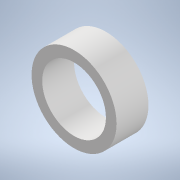
# Autodesk Inventor part: 3mmSpacer
Saved by Autodesk Inventor 2022 (Build 260153000, 153)
## iProperties
Created: 2023-09-19
Part Number: 3mmSpacer
Material: Generic
Document SubType Name: Modeling
Designer: THK
Density: 1 g/cm^3
Appearance: Default
Author: THK
Autodesk Inventor part; units mm, degrees
ref_plane "YZ Plane" through (0, 0, 0) normal (1, 0, 0) x (0, 1, 0)
ref_plane "XZ Plane" through (0, 0, 0) normal (0, 1, 0) x (-1, 0, 0)
ref_plane "XY Plane" through (0, 0, 0) normal (0, 0, 1) x (1, 0, 0)
sketch "Sketch1" plane through (0, 0, 0) normal (0, 0, 1) x (1, 0, 0)
  circle A0 centre (0, 0) radius 3
  circle A1 centre (0, 0) radius 4
  dimension "d0" = 6
  dimension "d1" = 8
  constraints: 2 centre point, 2 coincident
  measures "d0" diameter of A0
  measures "d1" diameter of A1
extrude "Extrusion1" add sketch "Sketch1" along normal blind 3
body "Solid1"
